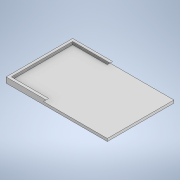
# Autodesk Inventor part: Mirror
Saved by Autodesk Inventor 2022.2 (Build 262287010, 287A)
## iProperties
Created: 2022-03-26
Part Number: Mirror
Material: Genérico
Document SubType Name: Modeling
Designer: mabel
Density: 1 g/cm^3
Appearance: Valor por defecto
Author: mabel
Autodesk Inventor part; units mm, degrees
ref_plane "YZ Plane" through (0, 0, 0) normal (1, 0, 0) x (0, 1, 0)
ref_plane "XZ Plane" through (0, 0, 0) normal (0, 1, 0) x (-1, 0, 0)
ref_plane "XY Plane" through (0, 0, 0) normal (0, 0, 1) x (1, 0, 0)
sketch "Boceto1" plane through (0, 0, 0) normal (0, 1, 0) x (-1, 0, 0)
  line L0 (-38, -25) -> (38, -25)
  line L1 (38, -25) -> (38, 25)
  line L2 (38, 25) -> (-38, 25)
  line L3 (-38, 25) -> (-38, -25)
  line L4 (-38, -25) -> (38, 25) construction
  line L5 (38, -25) -> (-38, 25) construction
  point P0 (0, 0)
  dimension "d0" = 76
  dimension "d1" = 50
  constraints: 12 end point, 2 midpoint, 2 parallel, 1 horizontal, 1 perpendicular
  measures "d0" distance of L2.end L1.end
  measures "d1" distance of L1.end L0.end
extrude "Extrusión1" add sketch "Boceto1" along normal blind 2
sketch "Boceto2" plane through (0, 2, 0) normal (0, 1, 0) x (1, 0, 0)
  line L0 (38, 25) -> (-38, 25) projected
  line L1 (-38, -25) -> (-10, -25)
  line L2 (-38, -25) -> (38, -25) projected
  line L3 (-38, -25) -> (-38, 25)
  line L4 (-38, 25) -> (-10, 25)
  line L5 (-10, 23) -> (-36, 23)
  line L6 (-36, 23) -> (-36, -23)
  line L7 (-36, -23) -> (-10, -23)
  line L8 (-10, 25) -> (-10, 23)
  line L9 (-10, -23) -> (-10, -25)
  point P0 (0, 0)
  point P1 (0, 25)
  dimension "d14" = 2
  constraints: 16 end point, 3 vertical, 2 point on line, 1 midpoint, 2 other
  measures "d14" distance between parallel lines of L3 L6
extrude "Extrusión4" add sketch "Boceto2" along normal blind 2
sketch "Boceto5" plane through (-38, 0, 25) normal (0, 0, 1) x (1, 0, 0)
  line L0 (28, 2) -> (28, 4) projected
  line L1 (28, 4) -> (28, 2)
  line L2 (76, 2) -> (28, 2) projected
  line L3 (28, 2) -> (30, 4)
  line L4 (28, 2) -> (32.2548, 2) construction
  line L5 (28, 4) -> (30, 4)
  point P0 (38, 0)
  constraints: 8 end point, 2 horizontal, 1 collinear
extrude "Extrusión5" add sketch "Boceto5" against normal blind 2
mirror "Simetría2" about plane through (0, 0, 0) normal (0, 0, 1) of "Extrusión5"
